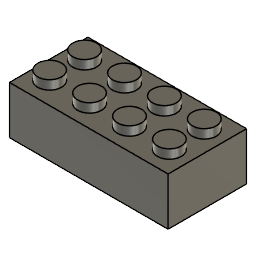
Lego Block (Autodesk Fusion 360 design; units mm, degrees)
part number: 2026-04-19-18-15-16-589
Autodesk Fusion 360 part; units mm, degrees
sketch "Sketch1" plane through (0, 0, 0) normal (0, 0, 1) x (1, 0, 0)
  line L0 (0, 0) -> (31.8055, 0)
  line L1 (31.8055, 0) -> (31.8055, -15.7354)
  line L2 (31.8055, -15.7354) -> (0, -15.7354)
  line L3 (0, -15.7354) -> (0, 0)
  constraint horizontal L0
  constraint vertical L1
  constraint horizontal L2
  constraint vertical L3
  constraint coincident L0.start L3.end
extrude "Extrude1" add sketch "Sketch1" along normal blind 9.6
sketch "Sketch2" plane through (0, 0, 9.6) normal (0, 0, 1) x (-1, 0, 0)
  line L0 (0, 15.7354) -> (-31.8055, 15.7354)
  line L1 (-31.8055, 15.7354) -> (-31.8055, 0)
  line L2 (-31.8055, 0) -> (0, 0)
  line L3 (0, 0) -> (0, 15.7354)
  circle A0 centre (-3.6827, 4.3523) radius 2.4
  dimension "d3" = 4.8
  measures "d3" diameter of A0
extrude "Extrude2" add sketch "Sketch2" along normal blind 1.8 contours A0
pattern_linear "R-Pattern1" count 4 spacing 8 along (1, 0, 0) of "Extrude2"
pattern_linear "R-Pattern2" count 2 spacing 7 along (0, -1, 0) of "Extrude2"
pattern_linear "R-Pattern3" count 4 spacing 8 along (1, 0, 0) of "R-Pattern2"
shell "Shell1" thickness 1.2 removed faces 1 at (10.6018, -10.4902, 0)
sketch "Sketch3" plane through (0, 0, 8.4) normal (0, 0, -1) x (1, 0, 0)
  line L0 (30.6055, 14.5354) -> (1.2, 14.5354)
  line L1 (1.2, 14.5354) -> (1.2, 1.2)
  line L2 (1.2, 1.2) -> (30.6055, 1.2)
  line L3 (30.6055, 1.2) -> (30.6055, 14.5354)
  circle A0 centre (3.6827, 4.3523) radius 1.2
  circle A1 centre (11.6827, 4.3523) radius 1.2
  circle A2 centre (19.6827, 4.3523) radius 1.2
  circle A3 centre (27.6827, 4.3523) radius 1.2
  circle A4 centre (3.6827, 11.3523) radius 1.2
  circle A5 centre (11.6827, 11.3523) radius 1.2
  circle A6 centre (19.6827, 11.3523) radius 1.2
  circle A7 centre (27.6827, 11.3523) radius 1.2
  circle A8 centre (7.2436, 7.8677) radius 3
  dimension "d19" = 6
  measures "d19" diameter of A8
extrude "Extrude3" add sketch "Sketch3" along normal blind 8 contours A8
pattern_linear "R-Pattern4" count 3 spacing 8.5 along (1, 0, 0) of "Extrude3"
